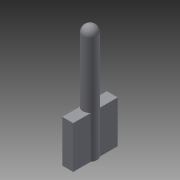
# Autodesk Inventor part: Dreidel Pole
Saved by Autodesk Inventor 2015 (Build 190159000, 159)
## iProperties
Created: 2018-05-10
Part Number: Dreidel Pole
Material: Generic
Document SubType Name: Modeling
Designer: Administrator
Density: 1 g/cm^3
Appearance: Default
Author: Administrator
Autodesk Inventor part; units mm, degrees
ref_plane "YZ Plane" through (0, 0, 0) normal (1, 0, 0) x (0, 1, 0)
ref_plane "XZ Plane" through (0, 0, 0) normal (0, 1, 0) x (-1, 0, 0)
ref_plane "XY Plane" through (0, 0, 0) normal (0, 0, 1) x (1, 0, 0)
sketch "Sketch1" plane through (0, 0, 0) normal (0, 1, 0) x (-1, 0, 0)
  line L0 (-1.2238, 7.2044) -> (3.6022, 7.2044)
  line L1 (3.6022, -12.6076) -> (-1.2238, -12.6076)
  line L2 (3.6022, 7.2044) -> (3.6022, -0.6381)
  line L3 (3.6022, -4.7651) -> (3.6022, -12.6076)
  line L4 (-1.2238, -12.6076) -> (-1.2238, -4.7651)
  line L5 (-1.2238, -0.6381) -> (-1.2238, 7.2044)
  arc A0 (-1.2238, -0.6381) -> (-1.2238, -4.7651) centre (1.1892, -2.7016) ccw
  arc A1 (3.6022, -4.7651) -> (3.6022, -0.6381) centre (1.1892, -2.7016) ccw
  circle A2 centre (1.1892, -2.7016) radius 3.175
  point P0 (0, 0)
  dimension "d0" = 19.812
  dimension "d1" = 4.826
  dimension "d3" = 9.906
  constraints: 12 end point, 5 parallel, 4 point on circle, 2 centre point, 2 perpendicular, 1 coincident, 1 horizontal, 3 other
  measures "d0" distance of L0.end L1.start
  measures "d1" distance of L0.start L0.end
  measures "d3" distance from line of L1 A0.centre
extrude "Extrusion1" add sketch "Sketch1" along normal blind 18.796 contours L0 L2 A2 L5 | A2 L3 L1 L4
extrude "Extrusion2" add sketch "Sketch1" along normal blind 50.8 contours A2 A1 A0
fillet "Fillet1" radius 3.175 1 edges at (1.9858, 50.8, -2.7016)
body "Solid1"
